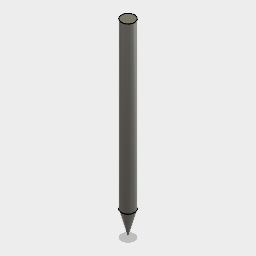
FPROJ_2 (Autodesk Fusion 360 design; units mm, degrees)
Autodesk Fusion 360 part; units mm, degrees
sketch "草图1" plane through (0, 0, 0) normal (1, 0, 0) x (0, 0, -1)
cylinder "圆柱体基本要素1" add diameter 8 height 100 placed x (1, 0, 0) y (0, 0, -1) z (0, 1, 0) at (0, 0, 0) makes body 1
sketch "草图3" plane through (0, 0, 0) normal (0, 0, 1) x (1, 0, 0)
  line L0 (0, 0) -> (4, 0)
  line L1 (4, 0) -> (0, -10)
  line L2 (0, -10) -> (0, 0)
  dimension "d3" = 4
  measures "d3" distance of L0.start L0.end
sketch "草图4" plane through (0, 0, 0) normal (0, 0, 1) x (1, 0, 0)
  line L0 (0, 0) -> (4, 0)
  line L1 (0, 0) -> (0, -15)
  line L2 (0, -15) -> (4, 0)
  dimension "d5" = 4
  dimension "d6" = 15
  measures "d5" distance of L0.start L0.end
  measures "d6" distance of L0.start L1.end
revolve "旋转2" add sketch "草图4" angle 360 about axis through (0, 0, 0) along (0, -1, 0) separate body makes body 2
combine "合并1" operation add target body 2 tool bodies 1
